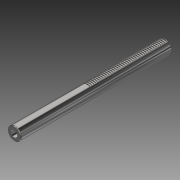
# Autodesk Inventor part: Weight_Shaft_Gear_Tube-01
Saved by Autodesk Inventor 2015 (Build 190159000, 159)
## iProperties
Created: 2015-01-18
Part Number: Weight_Shaft_Gear_Tube-01
Material: Generic
Document SubType Name: Modeling
Designer: Drew
Density: 1 g/cm^3
Appearance: Steel - Polished
Author: Drew
Autodesk Inventor part; units mm, degrees
ref_plane "YZ Plane" through (0, 0, 0) normal (1, 0, 0) x (0, 1, 0)
ref_plane "XZ Plane" through (0, 0, 0) normal (0, 1, 0) x (-1, 0, 0)
ref_plane "XY Plane" through (0, 0, 0) normal (0, 0, 1) x (1, 0, 0)
sketch "Sketch1" plane through (0, 0, 0) normal (0, 0, 1) x (1, 0, 0)
  circle A0 centre (0, 0) radius 3.175
  circle A1 centre (0, 0) radius 6.35
  dimension "d0" = 6.35
  dimension "d1" = 12.7
  constraints: 2 centre point, 2 coincident
  measures "d0" diameter of A0
  measures "d1" diameter of A1
extrude "Extrusion1" add sketch "Sketch1" along normal blind 146.05
chamfer "Chamfer1" distance 0.635 angle 45 2 edges at (-6.35, 0, 146.05) (-6.35, 0, 0)
sketch "Sketch2" plane through (0, 0, 0) normal (1, 0, 0) x (0, 1, 0)
  line L0 (6.35, 1.27) -> (5.842, 1.27)
  line L1 (5.842, 1.27) -> (5.842, 2.032)
  line L2 (5.842, 2.032) -> (6.35, 2.032)
  line L3 (6.35, 2.032) -> (6.35, 1.27)
  line L4 (5.715, 0) -> (-5.715, 0) projected
  line L5 (6.35, 145.415) -> (-6.35, 145.415) projected
  line L6 (6.35, 145.415) -> (6.35, 0.635)
  line L7 (-6.35, 0.635) -> (6.35, 0.635) projected
  point P0 (0, 0)
  point P1 (6.35, 1.651)
  dimension "d7" = 1.27
  dimension "d8" = 0.762
  dimension "d9" = 0.508
  constraints: 12 end point, 3 perpendicular, 1 horizontal, 1 midpoint, 1 point on line, 1 vertical
  measures "d7" distance between parallel lines of L4 L0
  measures "d8" distance of L2.end L0.start
  measures "d9" distance of L0.start L0.end
extrude "Extrusion2" cut sketch "Sketch2" along normal through all both and the other way through all
pattern_linear "Rectangular Pattern1" count 40 spacing 1.905 along (0, 0, 1) of "Extrusion2"
body "Solid1"
